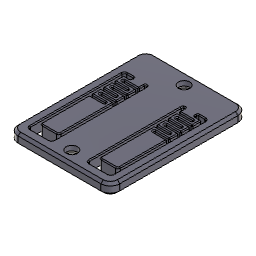
SSR DIN Rail Mount v1 (Autodesk Fusion 360 design; units mm, degrees)
Autodesk Fusion 360 part; units mm, degrees
note: some values were not read from the file. Set by a fixed rule: the direction of a hole.
sketch "Sketch1" plane through (0, 0, 0) normal (0, 0, 1) x (1, 0, 0)
  line L0 (21.5, 29) -> (21.5, -29)
  line L1 (21.5, -29) -> (-21.5, -29)
  line L2 (-21.5, -29) -> (-21.5, 29)
  line L3 (-21.5, 29) -> (21.5, 29)
  line L4 (0, -29) -> (0, 29) construction
  line L5 (-21.5, 0) -> (21.5, 0) construction
  point P0 (0, -23.75)
  point P1 (0, 23.75)
  dimension "d76" = 43
  dimension "d77" = 58
  dimension "d145" = 47.5
  constraint perpendicular L1 L2
  constraint perpendicular L2 L3
  constraint vertical L0
  constraint perpendicular L0 L3
  constraint midpoint L1 L4.start
  constraint midpoint L3 L4.end
  constraint midpoint L2 L5.start
  constraint midpoint L0 L5.end
  constraint coincident origin L4
  constraint coincident origin L5
  constraint coincident L4 P0
  constraint coincident L4 P1
  constraint symmetric L5 P0 P1
  measures "d76" distance of L1.end L0.end
  measures "d77" distance of L1 L3
  measures "d145" distance of P0 P1
extrude "Extrude5" add sketch "Sketch1" along normal blind 4.6
hole "Hole2" at (0, -23.75, 0) at (0, 23.75, 0) direction (0, 0, 1) diameter 4.8 depth 9.1 tip angle 180 countersink diameter 10 countersink angle 90
ref_plane "WorkPlane1" through (0, 0, 4.6) normal (0, 0, 1) x (1, 0, 0)
sketch "Sketch3" plane through (0, 0, 4.6) normal (0, 0, 1) x (1, 0, 0)
  line L0 (-17.5, 16) -> (-7.5, 16)
  line L1 (-7.5, 16) -> (-7.5, -24.8)
  line L2 (-7.5, -24.8) -> (-17.5, -24.8)
  line L3 (-17.5, -24.8) -> (-17.5, 16)
  line L4 (-8.5, 16) -> (-8.5, 13)
  line L5 (-8.5, 13) -> (-14.9, 13)
  line L6 (-14.9, 13) -> (-14.9, 12.2)
  line L7 (-14.9, 12.2) -> (-8.5, 12.2)
  line L8 (-8.5, 12.2) -> (-8.5, 8.2)
  line L9 (-8.5, 8.2) -> (-14.9, 8.2)
  line L10 (-14.9, 8.2) -> (-14.9, 7.4)
  line L11 (-14.9, 7.4) -> (-8.5, 7.4)
  line L12 (-8.5, 7.4) -> (-8.5, 3.4)
  line L13 (-8.5, 3.4) -> (-14.9, 3.4)
  line L14 (-14.9, 3.4) -> (-14.9, 2.6)
  line L15 (-14.9, 2.6) -> (-8.5, 2.6)
  line L16 (-8.5, 2.6) -> (-8.5, -20.8)
  line L17 (-13.5, 16) -> (-13.5, 14.6)
  line L18 (-13.5, 14.6) -> (-16.5, 14.6)
  line L19 (-16.5, 14.6) -> (-16.5, 10.6)
  line L20 (-16.5, 10.6) -> (-10.1, 10.6)
  line L21 (-10.1, 10.6) -> (-10.1, 9.8)
  line L22 (-10.1, 9.8) -> (-16.5, 9.8)
  line L23 (-16.5, 9.8) -> (-16.5, 5.8)
  line L24 (-16.5, 5.8) -> (-10.1, 5.8)
  line L25 (-10.1, 5.8) -> (-10.1, 5)
  line L26 (-10.1, 5) -> (-16.5, 5)
  line L27 (-16.5, 5) -> (-16.5, 1)
  line L28 (-16.5, 1) -> (-10.1, 1)
  line L29 (-10.1, 1) -> (-10.1, 0.2)
  line L30 (-10.1, 0.2) -> (-16.5, 0.2)
  line L31 (-16.5, 0.2) -> (-16.5, -20.8)
  line L32 (-16.5, -20.8) -> (-8.5, -20.8)
  line L33 (-14.9, 13) -> (-16.5, 13) construction
  line L34 (-14.9, 12.2) -> (-14.9, 10.6) construction
  line L35 (-10.1, 10.6) -> (-8.5, 10.6) construction
  line L36 (-10.1, 9.8) -> (-10.1, 8.2) construction
  line L37 (-14.9, 8.2) -> (-16.5, 8.2) construction
  line L38 (-14.9, 7.4) -> (-14.9, 5.8) construction
  line L39 (-10.1, 5.8) -> (-8.5, 5.8) construction
  line L40 (-10.1, 5) -> (-10.1, 3.4) construction
  line L41 (-14.9, 3.4) -> (-16.5, 3.4) construction
  line L42 (-14.9, 2.6) -> (-14.9, 1) construction
  line L43 (-10.1, 1) -> (-8.5, 1) construction
  line L44 (-13.5, 14.6) -> (-13.5, 13) construction
  line L45 (-16.5, -16) -> (-8.5, -16)
  line L46 (-12.5, -16) -> (-12.5, 16) construction
  line L47 (-17.5, 16) -> (-17.5, 28)
  line L48 (-17.5, 28) -> (-7.5, 28)
  line L49 (-7.5, 28) -> (-7.5, 16)
  line L50 (-21.5, -29) -> (-21.5, 29) construction
  line L51 (-21.5, 29) -> (21.5, 29) construction
  line L52 (21.5, 29) -> (21.5, -29) construction
  line L53 (-21.5, -29) -> (21.5, -29) construction
  line L54 (-21.5, 0) -> (21.5, 0) construction
  point P0 (-21.5, 29)
  point P1 (21.5, 29)
  point P2 (-21.5, -29)
  point P3 (-12.5, 0)
  dimension "d84" = 10
  dimension "d88" = 0.8
  dimension "d89" = 3
  dimension "d90" = 1
  dimension "d91" = 1
  dimension "d92" = 5
  dimension "d93" = 4
  dimension "d95" = 1.6
  dimension "d98" = 4.8
  dimension "d100" = 32
  dimension "d104" = 12
  dimension "d144" = 4
  constraint horizontal L0
  constraint vertical L1
  constraint horizontal L2
  constraint vertical L3
  constraint coincident L0 L4.start
  constraint perpendicular L0 L4
  constraint perpendicular L4 L5
  constraint perpendicular L5 L6
  constraint perpendicular L6 L7
  constraint perpendicular L7 L8
  constraint perpendicular L8 L9
  constraint perpendicular L9 L10
  constraint perpendicular L10 L11
  constraint perpendicular L11 L12
  constraint perpendicular L12 L13
  constraint perpendicular L13 L14
  constraint perpendicular L14 L15
  constraint perpendicular L15 L16
  constraint coincident L0 L17.start
  constraint perpendicular L0 L17
  constraint perpendicular L17 L18
  constraint perpendicular L18 L19
  constraint perpendicular L17 L20
  constraint perpendicular L20 L21
  constraint perpendicular L21 L22
  constraint perpendicular L22 L23
  constraint perpendicular L23 L24
  constraint perpendicular L24 L25
  constraint perpendicular L25 L26
  constraint perpendicular L26 L27
  constraint perpendicular L27 L28
  constraint perpendicular L28 L29
  constraint perpendicular L27 L30
  constraint perpendicular L31 L32
  constraint collinear L27 L31
  constraint collinear L23 L27
  constraint collinear L19 L23
  constraint collinear L4 L8
  constraint collinear L8 L12
  constraint collinear L12 L16
  constraint coincident L19 L33.end
  constraint perpendicular L19 L33
  constraint coincident L20 L34.end
  constraint perpendicular L20 L34
  constraint coincident L8 L35.end
  constraint perpendicular L8 L35
  constraint coincident L9 L36.end
  constraint perpendicular L9 L36
  constraint perpendicular L10 L37
  constraint coincident L23 L37.end
  constraint coincident L24 L38.end
  constraint perpendicular L24 L38
  constraint coincident L12 L39.end
  constraint perpendicular L12 L39
  constraint coincident L13 L40.end
  constraint perpendicular L13 L40
  constraint coincident L27 L41.end
  constraint perpendicular L27 L41
  constraint coincident L28 L42.end
  constraint perpendicular L28 L42
  constraint coincident L16 L43.end
  constraint perpendicular L16 L43
  constraint equal L34 L35
  constraint equal L36 L37
  constraint equal L37 L38
  constraint equal L38 L39
  constraint equal L39 L40
  constraint equal L40 L41
  constraint equal L41 L42
  constraint equal L42 L43
  constraint equal L6 L21
  constraint equal L10 L21
  constraint equal L10 L25
  constraint equal L14 L25
  constraint equal L14 L29
  constraint equal L35 L36
  constraint equal L33 L34
  constraint coincident L5 L44.end
  constraint perpendicular L5 L44
  constraint equal L33 L44
  constraint coincident L31 L45.start
  constraint coincident L16 L45.end
  constraint perpendicular L16 L45
  constraint midpoint L45 L46.start
  constraint midpoint L0 L46.end
  constraint midpoint L46 P3
  constraint perpendicular L0 L47
  constraint perpendicular L47 L48
  constraint perpendicular L48 L49
  constraint coincident P2 L50.start
  constraint coincident P0 L50.end
  constraint coincident P1 L51.end
  constraint perpendicular L51 L52
  constraint perpendicular L50 L53
  constraint coincident L52.end L53.end
  constraint midpoint L50 L54.start
  constraint midpoint L52 L54.end
  constraint coincident P3 L54
  measures "d84" distance of L1.end L2.end
  measures "d88" distance of L5 L7
  measures "d89" distance of L4.start L4.end
  measures "d90" distance of L3 L19
  measures "d91" distance of L1 L8
  measures "d92" distance of L4 L17
  measures "d93" distance of L2 L32
  measures "d95" distance of L5 L18
  measures "d98" distance of L32 L45
  measures "d100" distance of L0 L45
  measures "d104" distance of L0.start L47.end
  measures "d144" distance of L3 L50
extrude "Extrude6" cut sketch "Sketch3" against normal through all contours L0 L1 L2 L3 L4 L5 L6 L7 L8 L9 L10 L11 L12 L13 L14 L15 L16 L17 L18 L19 L20 L21 L22 L23 L24 L25 L26 L27 L28 L29 L30 L31 L32
extrude "Extrude7" add sketch "Sketch3" against normal blind 3 from surface at -4.6 contours L0 L47 L48 L49 | L16 L31 L32 L45
ref_plane "WorkPlane2" through (-17.5, 22, -1.5) normal (-1, 0, 0) x (0, 1, 0)
sketch "Sketch4" plane through (-17.5, 0, 0) normal (-1, 0, 0) x (0, -1, 0)
  line L0 (-16, -3) -> (-16, 0) construction
  line L1 (-16, 0) -> (-28, 0) construction
  line L2 (-28, 0) -> (-28, -3) construction
  line L3 (-28, -3) -> (-16, -3) construction
  line L4 (20.8, -3) -> (16, -3) construction
  line L5 (16, -3) -> (16, 0) construction
  line L6 (20.8, -3) -> (20.8, 0) construction
  line L7 (20.8, 0) -> (16, 0) construction
  line L8 (17.4, 0) -> (17.4, -0.75)
  line L9 (17.4, -0.75) -> (16, -2.15)
  line L10 (16, -2.15) -> (16, 0)
  line L11 (17.4, 0) -> (16, 0)
  line L12 (-16, 0) -> (-17.4, 0)
  line L13 (-17.4, 0) -> (-17.4, -0.75)
  line L14 (-17.4, -0.75) -> (-16, -2.15)
  line L15 (-16, -2.15) -> (-16, 0)
  point P0 (16, 0)
  point P1 (-16, -3)
  point P2 (-28, -3)
  point P3 (-16, 0)
  point P4 (-28, 0)
  point P5 (16, -3)
  point P6 (20.8, -3)
  dimension "d106" = 0.75
  dimension "d107" = 45
  dimension "d108" = 1.4
  dimension "d109" = 135
  constraint coincident P1 L0.start
  constraint coincident P3 L0.end
  constraint coincident P4 L1.end
  constraint coincident P2 L2.end
  constraint coincident P0 L5.end
  constraint vertical L6
  constraint perpendicular L6 L7
  constraint coincident L7 L8.start
  constraint perpendicular L7 L8
  constraint coincident L5 L9.end
  constraint coincident L1 L12.end
  constraint perpendicular L0 L12
  constraint perpendicular L1 L13
  constraint perpendicular L12 L15
  constraint equal L8 L13
  constraint equal L11 L12
  measures "d106" distance of L8.start L8.end
  measures "d107" angle of L8 L9
  measures "d108" distance of P0 L8.start
  measures "d109" angle of L13 L14
extrude "Extrude8" cut sketch "Sketch4" against normal through all
fillet "Fillet3" radius 1 20 edges at (-16.5, -20.8, 0.8) (-8.5, -20.8, 0.8) (-7.5, -24.8, 2.3) (-17.5, -24.8, 2.3) (-17.5, 16, 2.3) (-7.5, 16, 2.3) (-17.5, 28, -1.5) (-7.5, 28, -1.5) (-17.5, 17.4, -0.375) (-17.5, 16, -2.575) (-17.5, 16.7, -1.45) (-7.5, 17.4, -0.375) (-7.5, 16.7, -1.45) (-7.5, 16, -2.575) (-16.5, -17.4, -0.375) (-16.5, -16.7, -1.45) (-16.5, -16, -2.575) (-8.5, -17.4, -0.375) (-8.5, -16.7, -1.45) (-8.5, -16, -2.575)
fillet "Fillet4" radius 0.4 28 edges at (-10.1, 0.2, 2.3) (-10.1, 1, 2.3) (-16.5, 0.2, 2.3) (-16.5, 1, 2.3) (-14.9, 2.6, 2.3) (-14.9, 3.4, 2.3) (-16.5, 5.8, 2.3) (-16.5, 5, 2.3) (-8.5, 3.4, 2.3) (-8.5, 2.6, 2.3) (-10.1, 5, 2.3) (-10.1, 5.8, 2.3) (-8.5, 7.4, 2.3) (-8.5, 8.2, 2.3) (-14.9, 7.4, 2.3) (-14.9, 8.2, 2.3) (-16.5, 9.8, 2.3) (-16.5, 10.6, 2.3) (-10.1, 9.8, 2.3) (-10.1, 10.6, 2.3) (-8.5, 12.2, 2.3) (-8.5, 13, 2.3) (-8.5, 16, 2.3) (-13.5, 16, 2.3) (-13.5, 14.6, 2.3) (-16.5, 14.6, 2.3) (-14.9, 12.2, 2.3) (-14.9, 13, 2.3)
mirror "Mirror2" about plane through (0, 0, 0) normal (1, 0, 0) of "Extrude6", "Extrude7", "Extrude8", "Fillet3", "Fillet4"
fillet "Fillet5" radius 4 4 edges at (-21.5, -29, 2.3) (21.5, -29, 2.3) (-21.5, 29, 2.3) (21.5, 29, 2.3)
chamfer "Chamfer3" distance 1 angle 45 16 edges at (21.5, 0, 0) (20.3284, -27.8284, 0) (0, -29, 0) (-20.3284, -27.8284, 0) (-21.5, 0, 0) (-20.3284, 27.8284, 0) (0, 29, 0) (20.3284, 27.8284, 0) (21.5, 0, 4.6) (20.3284, 27.8284, 4.6) (0, 29, 4.6) (-20.3284, 27.8284, 4.6) (-21.5, 0, 4.6) (-20.3284, -27.8284, 4.6) (0, -29, 4.6) (20.3284, -27.8284, 4.6)
chamfer "Chamfer4" distance 0.4 angle 45 246 edges at (-7.5, 22, -3) (-7.7929, 16.2929, -3) (-12.5, 16, -3) (-17.2071, 16.2929, -3) (-17.5, 22, -3) (-17.2071, 27.7071, -3) (-12.5, 28, -3) (-7.7929, 27.7071, -3) (7.5, 22, -3) (7.7929, 27.7071, -3) (12.5, 28, -3) (17.2071, 27.7071, -3) (17.5, 22, -3) (17.2071, 16.2929, -3) (12.5, 16, -3) (7.7929, 16.2929, -3) (-8.5, -18.4, -3) (-8.7929, -20.5071, -3) (-12.5, -20.8, -3) (-16.2071, -20.5071, -3) (-16.5, -18.4, -3) (-16.2071, -16.2929, -3) (-12.5, -16, -3) (-8.7929, -16.2929, -3) (8.5, -18.4, -3) (8.7929, -16.2929, -3) (12.5, -16, -3) (16.2071, -16.2929, -3) (16.5, -18.4, -3) (16.2071, -20.5071, -3) (12.5, -20.8, -3) (8.7929, -20.5071, -3) (16.5, 7.8, 0) (16.3828, 5.9172, 0) (13.3, 5.8, 0) (10.1, 5.4, 0) (13.3, 5, 0) (16.3828, 4.8828, 0) (16.5, 3, 0) (16.3828, 1.1172, 0) (13.3, 1, 0) (10.1, 0.6, 0) (13.3, 0.2, 0) (16.3828, 0.0828, 0) (16.5, -9.3, 0) (8.5, -8.1, 0) (8.6172, 2.4828, 0) (11.7, 2.6, 0) (14.9, 3, 0) (11.7, 3.4, 0) (8.6172, 3.5172, 0) (8.5, 5.4, 0) (8.6172, 7.2828, 0) (11.7, 7.4, 0) (14.9, 7.8, 0) (11.7, 8.2, 0) (8.6172, 8.3172, 0) (8.5, 10.2, 0) (8.6172, 12.0828, 0) (11.7, 12.2, 0) (14.9, 12.6, 0) (11.7, 13, 0) (8.6172, 13.1172, 0) (8.5, 14.4236, 0) (8.2633, 15.8124, 0) (7.5871, 15.4082, 0) (7.5, -4.4, 0) (7.7929, -24.5071, 0) (12.5, -24.8, 0) (17.2071, -24.5071, 0) (17.5, -4.4, 0) (17.2071, 15.7071, 0) (15.2, 16, 0) (13.6172, 15.8828, 0) (13.5, 15.3, 0) (13.6172, 14.7172, 0) (15, 14.6, 0) (16.3828, 14.4828, 0) (16.5, 12.6, 0) (16.3828, 10.7172, 0) (13.3, 10.6, 0) (10.1, 10.2, 0) (13.3, 9.8, 0) (16.3828, 9.6828, 0) (17.5, -4.4, 4.6) (17.2071, -24.5071, 4.6) (12.5, -24.8, 4.6) (7.7929, -24.5071, 4.6) (7.5, -4.4, 4.6) (7.5871, 15.4082, 4.6) (8.2633, 15.8124, 4.6) (8.5, 14.4236, 4.6) (8.6172, 13.1172, 4.6) (11.7, 13, 4.6) (14.9, 12.6, 4.6) (11.7, 12.2, 4.6) (8.6172, 12.0828, 4.6) (8.5, 10.2, 4.6) (8.6172, 8.3172, 4.6) (11.7, 8.2, 4.6) (14.9, 7.8, 4.6) (11.7, 7.4, 4.6) (8.6172, 7.2828, 4.6) (8.5, 5.4, 4.6) (8.6172, 3.5172, 4.6) (11.7, 3.4, 4.6) (14.9, 3, 4.6) (11.7, 2.6, 4.6) (8.6172, 2.4828, 4.6) (8.5, -8.8, 4.6) (8.7929, -20.5071, 4.6) (12.5, -20.8, 4.6) (16.2071, -20.5071, 4.6) (16.5, -10, 4.6) (16.3828, 0.0828, 4.6) (13.3, 0.2, 4.6) (10.1, 0.6, 4.6) (13.3, 1, 4.6) (16.3828, 1.1172, 4.6) (16.5, 3, 4.6) (16.3828, 4.8828, 4.6) (13.3, 5, 4.6) (10.1, 5.4, 4.6) (13.3, 5.8, 4.6) (16.3828, 5.9172, 4.6) (16.5, 7.8, 4.6) (16.3828, 9.6828, 4.6) (13.3, 9.8, 4.6) (10.1, 10.2, 4.6) (13.3, 10.6, 4.6) (16.3828, 10.7172, 4.6) (16.5, 12.6, 4.6) (16.3828, 14.4828, 4.6) (15, 14.6, 4.6) (13.6172, 14.7172, 4.6) (13.5, 15.3, 4.6) (13.6172, 15.8828, 4.6) (15.2, 16, 4.6) (17.2071, 15.7071, 4.6) (-17.5, -4.4, 4.6) (-17.2071, 15.7071, 4.6) (-15.2, 16, 4.6) (-13.6172, 15.8828, 4.6) (-13.5, 15.3, 4.6) (-13.6172, 14.7172, 4.6) (-15, 14.6, 4.6) (-16.3828, 14.4828, 4.6) (-16.5, 12.6, 4.6) (-16.3828, 10.7172, 4.6) (-13.3, 10.6, 4.6) (-10.1, 10.2, 4.6) (-13.3, 9.8, 4.6) (-16.3828, 9.6828, 4.6) (-16.5, 7.8, 4.6) (-16.3828, 5.9172, 4.6) (-13.3, 5.8, 4.6) (-10.1, 5.4, 4.6) (-13.3, 5, 4.6) (-16.3828, 4.8828, 4.6) (-16.5, 3, 4.6) (-16.3828, 1.1172, 4.6) (-13.3, 1, 4.6) (-10.1, 0.6, 4.6) (-13.3, 0.2, 4.6) (-16.3828, 0.0828, 4.6) (-16.5, -10, 4.6) (-16.2071, -20.5071, 4.6) (-12.5, -20.8, 4.6) (-8.7929, -20.5071, 4.6) (-8.5, -8.8, 4.6) (-8.6172, 2.4828, 4.6) (-11.7, 2.6, 4.6) (-14.9, 3, 4.6) (-11.7, 3.4, 4.6) (-8.6172, 3.5172, 4.6) (-8.5, 5.4, 4.6) (-8.6172, 7.2828, 4.6) (-11.7, 7.4, 4.6) (-14.9, 7.8, 4.6) (-11.7, 8.2, 4.6) (-8.6172, 8.3172, 4.6) (-8.5, 10.2, 4.6) (-8.6172, 12.0828, 4.6) (-11.7, 12.2, 4.6) (-14.9, 12.6, 4.6) (-11.7, 13, 4.6) (-8.6172, 13.1172, 4.6) (-8.5, 14.4236, 4.6) (-8.2633, 15.8124, 4.6) (-7.5871, 15.4082, 4.6) (-7.5, -4.4, 4.6) (-7.7929, -24.5071, 4.6) (-12.5, -24.8, 4.6) (-17.2071, -24.5071, 4.6) (-17.5, -4.4, 0) (-17.2071, -24.5071, 0) (-12.5, -24.8, 0) (-7.7929, -24.5071, 0) (-7.5, -4.4, 0) (-7.5871, 15.4082, 0) (-8.2633, 15.8124, 0) (-8.5, 14.4236, 0) (-8.6172, 13.1172, 0) (-11.7, 13, 0) (-14.9, 12.6, 0) (-11.7, 12.2, 0) (-8.6172, 12.0828, 0) (-8.5, 10.2, 0) (-8.6172, 8.3172, 0) (-11.7, 8.2, 0) (-14.9, 7.8, 0) (-11.7, 7.4, 0) (-8.6172, 7.2828, 0) (-8.5, 5.4, 0) (-8.6172, 3.5172, 0) (-11.7, 3.4, 0) (-14.9, 3, 0) (-11.7, 2.6, 0) (-8.6172, 2.4828, 0) (-8.5, -8.1, 0) (-16.5, -9.3, 0) (-16.3828, 0.0828, 0) (-13.3, 0.2, 0) (-10.1, 0.6, 0) (-13.3, 1, 0) (-16.3828, 1.1172, 0) (-16.5, 3, 0) (-16.3828, 4.8828, 0) (-13.3, 5, 0) (-10.1, 5.4, 0) (-13.3, 5.8, 0) (-16.3828, 5.9172, 0) (-16.5, 7.8, 0) (-16.3828, 9.6828, 0) (-13.3, 9.8, 0) (-10.1, 10.2, 0) (-13.3, 10.6, 0) (-16.3828, 10.7172, 0) (-16.5, 12.6, 0) (-16.3828, 14.4828, 0) (-15, 14.6, 0) (-13.6172, 14.7172, 0) (-13.5, 15.3, 0) (-13.6172, 15.8828, 0) (-15.2, 16, 0) (-17.2071, 15.7071, 0)
named bodies: "LRS-100-5 DIN Rail Mount"
